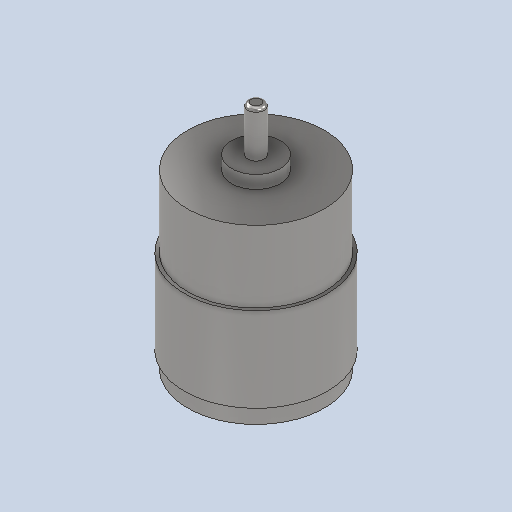
# Autodesk Inventor part: rs735
Saved by Autodesk Inventor 2025.1 (Build 291241000, 241)
## iProperties
Created: 2023-12-06
Part Number: rs735
Material: ステンレス鋼
Document SubType Name: Modeling
Designer: fhbdh
Density: 8 g/cm^3
Appearance: 半つや出し
Author: fhbdh
Autodesk Inventor part; units mm, degrees
ref_plane "YZ Plane" through (0, 0, 0) normal (1, 0, 0) x (0, 1, 0)
ref_plane "XZ Plane" through (0, 0, 0) normal (0, 1, 0) x (-1, 0, 0)
ref_plane "XY Plane" through (0, 0, 0) normal (0, 0, 1) x (1, 0, 0)
sketch "スケッチ1" plane through (0, 0, 0) normal (0, 1, 0) x (-1, 0, 0)
  circle A0 centre (0, 0) radius 21
  dimension "d0" = 42
  constraints: 1 centre point, 1 coincident
  measures "d0" diameter of A0
extrude "押し出し1" add sketch "スケッチ1" along normal blind 5
sketch "スケッチ2" plane through (0, 5, 0) normal (0, 1, 0) x (1, 0, 0)
  circle A0 centre (0, 0) radius 22
  dimension "d3" = 44
  constraints: 1 centre point, 1 coincident
  measures "d3" diameter of A0
extrude "押し出し2" add sketch "スケッチ2" along normal blind 26
sketch "スケッチ3" plane through (0, 31, 0) normal (0, 1, 0) x (1, 0, 0)
  circle A0 centre (0, 0) radius 21
  dimension "d6" = 42
  constraints: 1 centre point, 1 coincident
  measures "d6" diameter of A0
extrude "押し出し3" add sketch "スケッチ3" along normal blind 22
sketch "スケッチ4" plane through (0, 0, 0) normal (0, -1, 0) x (1, 0, 0)
  circle A0 centre (0, 0) radius 7.5
  dimension "d9" = 15
  constraints: 1 centre point, 1 coincident
  measures "d9" diameter of A0
extrude "押し出し4" add sketch "スケッチ4" along normal blind 4
sketch "スケッチ5" plane through (0, -4, 0) normal (0, -1, 0) x (1, 0, 0)
  circle A0 centre (0, 0) radius 2.5
  dimension "d12" = 5
  constraints: 1 centre point, 1 coincident
  measures "d12" diameter of A0
extrude "押し出し5" add sketch "スケッチ5" along normal blind 7
sketch "スケッチ6" plane through (0, 53, 0) normal (0, 1, 0) x (1, 0, 0)
  circle A0 centre (0, 0) radius 7.5
  dimension "d15" = 15
  constraints: 1 centre point, 1 coincident
  measures "d15" diameter of A0
extrude "押し出し6" add sketch "スケッチ6" along normal blind 4
sketch "スケッチ7" plane through (0, 57, 0) normal (0, 1, 0) x (1, 0, 0)
  circle A0 centre (0, 0) radius 2.5
  dimension "d18" = 5
  constraints: 1 centre point, 1 coincident
  measures "d18" diameter of A0
extrude "押し出し7" add sketch "スケッチ7" along normal blind 14
sketch "スケッチ8" plane through (0, 0, 0) normal (0, -1, 0) x (1, 0, 0)
  circle A0 centre (14.5, 0) radius 2
  circle A1 centre (0, 0) radius 7.5 projected
  line L0 (0, 0) -> (21, 0) construction
  circle A2 centre (0, 0) radius 21 projected
  circle A3 centre (-14.5, 0) radius 2
  dimension "d21" = 4
  dimension "d24" = 360
  dimension "d26" = 29
  constraints: 2 centre point, 2 end point, 1 horizontal, 1 horizontal alignment, 1 point on line, 6 other
  measures "d21" diameter of A0
  measures "d26" distance of A3.centre A0.centre
extrude "押し出し8" cut sketch "スケッチ8" against normal blind 5 contours A0 | A3
fillet "フィレット1" radius 1 2 edges at (-2.5, -11, 0) (-2.5, 71, 0)
